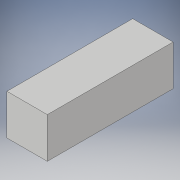
# Autodesk Inventor part: 1-Battery-Case
Saved by Autodesk Inventor 2019 (Build 230136000, 136)
## iProperties
Created: 2018-11-25
Part Number: 1-Battery-Case
Material: Generic
Document SubType Name: Modeling
Designer: lateSWE
Density: 1 g/cm^3
Appearance: Default
Author: lateSWE
Autodesk Inventor part; units mm, degrees
ref_plane "YZ Plane" through (0, 0, 0) normal (1, 0, 0) x (0, 1, 0)
ref_plane "XZ Plane" through (0, 0, 0) normal (0, 1, 0) x (-1, 0, 0)
ref_plane "XY Plane" through (0, 0, 0) normal (0, 0, 1) x (1, 0, 0)
sketch "Sketch1" plane through (0, 0, 0) normal (0, 0, 1) x (1, 0, 0)
  line L0 (0, 0) -> (22.5, 0)
  line L1 (22.5, 0) -> (22.5, 22.5)
  line L2 (22.5, 22.5) -> (0, 22.5)
  line L3 (0, 22.5) -> (0, 0)
  line L4 (0, 0) -> (20.5, 0)
  line L5 (20.5, 0) -> (20.5, 2)
  line L6 (20.5, 2) -> (0, 2)
  line L7 (0, 2) -> (0, 0)
  line L8 (22.5, 0) -> (20.5, 0)
  line L9 (20.5, 0) -> (20.5, 20.5)
  line L10 (20.5, 20.5) -> (22.5, 20.5)
  line L11 (22.5, 20.5) -> (22.5, 0)
  line L12 (22.5, 22.5) -> (2, 22.5)
  line L13 (2, 22.5) -> (2, 20.5)
  line L14 (2, 20.5) -> (22.5, 20.5)
  line L15 (22.5, 20.5) -> (22.5, 22.5)
  line L16 (0, 22.5) -> (2, 22.5)
  line L17 (2, 22.5) -> (2, 2)
  line L18 (2, 2) -> (0, 2)
  line L19 (0, 2) -> (0, 22.5)
  line L20 (2, 2) -> (20.5, 2)
  line L21 (20.5, 2) -> (20.5, 20.5)
  line L22 (20.5, 20.5) -> (2, 20.5)
  line L23 (2, 20.5) -> (2, 2)
  dimension "d0" = 22.5
  dimension "d1" = 22.5
  dimension "d2" = 20.5
  dimension "d3" = 2
  dimension "d4" = 2
  dimension "d5" = 20.5
  dimension "d6" = 20.5
  dimension "d7" = 2
  dimension "d8" = 2
  dimension "d9" = 20.5
  dimension "d10" = 18.5
  dimension "d11" = 18.5
  constraints: 48 end point, 12 parallel, 6 horizontal, 6 perpendicular
  measures "d0" distance of L2.end L1.end
  measures "d1" distance of L1.end L0.end
  measures "d2" distance of L6.end L5.end
  measures "d3" distance of L5.end L4.end
  measures "d4" distance of L9.end L10.end
  measures "d5" distance of L8.end L9.end
  measures "d6" distance of L14.end L13.end
  measures "d7" distance of L13.end L12.end
  measures "d8" distance of L17.end L18.end
  measures "d9" distance of L16.end L17.end
  measures "d10" distance of L22.end L9.end
  measures "d11" distance of L9.end L20.end
extrude "Extrusion1" add sketch "Sketch1" along normal blind 69
sketch "Sketch2" plane through (0, 0, 0) normal (0, -1, 0) x (1, 0, 0)
  line L0 (0, 69) -> (22.5, 69) projected
  line L1 (22.5, 69) -> (20.5, 69)
  line L2 (20.5, 69) -> (20.5, 2)
  line L3 (20.5, 2) -> (22.5, 2)
  line L4 (22.5, 2) -> (22.5, 69)
  line L5 (20.5, 2) -> (2, 2)
  line L6 (2, 2) -> (2, 68)
  line L7 (2, 68) -> (20.5, 68)
  line L8 (20.5, 68) -> (20.5, 2)
  point P0 (0, 0)
  dimension "d14" = 2
  dimension "d15" = 67
  dimension "d16" = 18.5
  dimension "d17" = 66
  constraints: 16 end point, 4 parallel, 2 horizontal, 2 perpendicular
  measures "d14" distance of L3.end L2.end
  measures "d15" distance of L2.end L1.end
  measures "d16" distance of L6.end L7.end
  measures "d17" distance of L5.end L6.end
extrude "Extrusion2" cut sketch "Sketch2" against normal blind 18.5 contours L2 L5 L6 L7
sketch "Sketch3" plane through (0, 0, 69) normal (0, 0, 1) x (1, 0, 0)
  line L0 (22.5, 22.5) -> (0, 22.5) projected
  line L1 (0, 0) -> (22.5, 0) projected
  line L2 (0, 22.5) -> (22.5, 22.5)
  line L3 (22.5, 22.5) -> (22.5, 0)
  line L4 (22.5, 0) -> (0, 0)
  line L5 (0, 0) -> (0, 22.5)
  dimension "d20" = 22.5
  dimension "d21" = 22.5
  constraints: 8 end point, 2 parallel, 1 horizontal, 1 perpendicular
  measures "d20" distance of L1.end L4.end
  measures "d21" distance of L2.end L1.end
extrude "Extrusion3" add sketch "Sketch3" along normal blind 1
sketch "Sketch4" plane through (0, 18.5, 0) normal (0, -1, 0) x (1, 0, 0)
  point P0 (0, 0)
sketch "Sketch5" plane through (0, 18.5, 0) normal (0, -1, 0) x (1, 0, 0)
  line L0 (20.5, 2) -> (2, 2) projected
  line L1 (20.5, 68) -> (20.5, 2) projected
  line L2 (2, 2) -> (20.5, 2)
  line L3 (20.5, 2) -> (20.5, 68)
  line L4 (20.5, 68) -> (2, 68)
  line L5 (2, 68) -> (2, 2)
  point P0 (0, 0)
  dimension "d24" = 18.5
  dimension "d25" = 66
  constraints: 8 end point, 2 parallel, 1 horizontal, 1 perpendicular
  measures "d24" distance of L4.end L1.start
  measures "d25" distance of L1.start L2.end
extrude "Extrusion4" cut sketch "Sketch5" against normal blind 2
body "Solid1"
